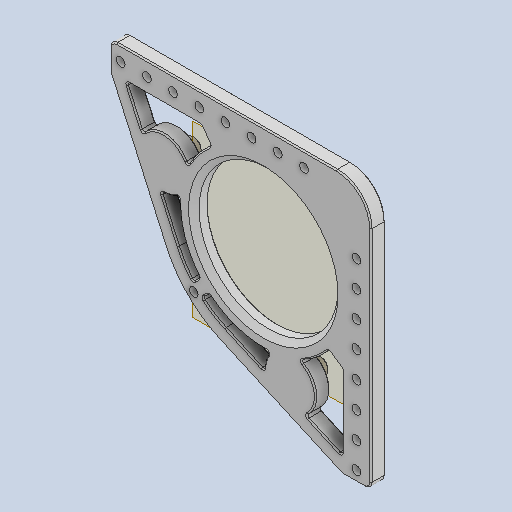
# Autodesk Inventor part: lower_plate
Saved by Autodesk Inventor 2022 (Build 260153000, 153)
## iProperties
Created: 2022-03-16
Part Number: lower_plate
Material: Generic
Document SubType Name: Modeling
Designer: zac-h
Density: 1 g/cm^3
Appearance: Default
Author: zac-h
## iProperties of the stored document lower_plate_3DPrint.ipt
Created: 2022-03-17
Part Number: lower_plate_3DPrint
Material: Generic
Document SubType Name: Modeling
Designer: zac-h
Density: 1 g/cm^3
Appearance: Default
Author: zac-h
Autodesk Inventor part; units mm, degrees
ref_plane "YZ Plane" through (0, 0, 0) normal (1, 0, 0) x (0, 1, 0)
ref_plane "XZ Plane" through (0, 0, 0) normal (0, 1, 0) x (-1, 0, 0)
ref_plane "XY Plane" through (0, 0, 0) normal (0, 0, 1) x (1, 0, 0)
ref_plane "Work Plane1" through (0, 0, 3) normal (0, 0, 1) x (1, 0, 0)
sketch "Sketch1" plane through (0, 0, 3) normal (0, 0, 1) x (1, 0, 0)
  circle A0 centre (-0.1388, 10.4389) radius 38.025 construction
  circle A1 centre (-0.1388, 10.4389) radius 33.675
  line L0 (41.1362, 10.4389) -> (-0.1388, 10.4389) construction
  circle A2 centre (-0.1388, 10.4389) radius 52.145
  line L1 (-0.1388, 62.5839) -> (-74.3588, 62.5839)
  line L2 (-74.3588, 62.5839) -> (-74.3588, 48.6139)
  line L3 (-74.3588, 48.6139) -> (-35.6602, 48.6139)
  line L4 (-74.3588, 55.5989) -> (45.0212, 55.5989) construction
  line L5 (45.0212, 55.5989) -> (-0.1388, 10.4389) construction
  circle A3 centre (-31.1788, 55.5989) radius 2.132
  circle A4 centre (-43.8788, 55.5989) radius 2.132
  circle A5 centre (-56.5788, 55.5989) radius 2.132
  circle A6 centre (-69.2788, 55.5989) radius 2.132
  line L6 (52.0062, 10.4389) -> (52.0062, -63.7811)
  line L7 (52.0062, -63.7811) -> (38.0362, -63.7811)
  line L8 (38.0362, -63.7811) -> (38.0362, -25.0825)
  circle A7 centre (45.0212, -20.6011) radius 2.132
  circle A8 centre (45.0212, -33.3011) radius 2.132
  circle A9 centre (45.0212, -46.0011) radius 2.132
  circle A10 centre (45.0212, -58.7011) radius 2.132
  line L9 (-47.7328, -10.8663) -> (-74.3588, 48.6139)
  line L10 (-21.444, -37.1551) -> (38.0362, -63.7811)
  circle A11 centre (-0.1388, 10.4389) radius 38.175 construction
  circle A12 centre (35.3403, 45.9179) radius 12 construction
  circle A13 centre (35.3403, 45.9179) radius 15
  line L11 (35.3403, 62.5839) -> (-0.1388, 62.5839)
  circle A14 centre (35.3403, 45.9179) radius 3.95
  circle A15 centre (-18.4788, 55.5989) radius 2.132
  circle A16 centre (-5.7788, 55.5989) radius 2.132
  circle A17 centre (6.9212, 55.5989) radius 2.132
  circle A18 centre (19.6212, 55.5989) radius 2.132
  circle A19 centre (45.0212, -7.9011) radius 2.132
  circle A20 centre (45.0212, 4.7989) radius 2.132
  circle A21 centre (45.0212, 17.4989) radius 2.132
  circle A22 centre (45.0212, 30.1989) radius 2.132
  circle A23 centre (35.3403, 45.9179) radius 16.6659
  line L12 (-35.6602, 48.6139) -> (12.0833, 48.6139) construction
  line L13 (52.0062, 45.9179) -> (52.0062, 10.4389)
  circle A24 centre (-33.8359, -23.2582) radius 2.132
  line L14 (-33.8359, -23.2582) -> (-37.0109, -26.4332) construction
  point P0 (0, 0)
  point P1 (24.5699, 56.3582)
  point P2 (45.7805, 35.1475)
  dimension "d0" = 4.35
  dimension "d11" = 13.97
  dimension "d12" = 45
  dimension "d13" = 4.264
  dimension "d14" = 76.2
  dimension "d17" = 12.7
  dimension "d23" = 119.38
  dimension "d47" = 0.15
  dimension "d48" = 24
  dimension "d49" = 30
  dimension "d50" = 7.9
  dimension "d91" = 12.7
  dimension "d96" = 4.264
  dimension "d99" = 3.175
  constraints: 30 end point, 24 centre point, 12 symmetric about line, 8 point on circle, 7 horizontal, 7 tangent, 5 coincident, 3 point on line, 2 perpendicular, 1 collinear, 1 midpoint, 22 other
  measures "d0" radial gap between concentric circles of A0 A1
  measures "d11" distance of L1.end L2.end
  measures "d12" angle of L0 L5
  measures "d13" diameter of A3
  measures "d14" distance of A3.centre L4.end
  measures "d17" distance of A3.centre A4.centre
  measures "d23" distance of L4.start L4.end
  measures "d47" radial gap between concentric circles of A0 A11
  measures "d48" diameter of A12
  measures "d49" diameter of A13
  measures "d50" diameter of A14
  measures "d91" distance of A3.centre A15.centre
  measures "d96" diameter of A24
  measures "d99" horizontal distance of L14.start L14.end
extrude "Extrusion1" add sketch "Sketch1" along normal blind 7 contours A1 A23 A22 A2 A18 | A1 A23 A18 A2 A13 A22 | A23 L13 A2 | A2 A13 A23 | A2 L11 A23 | L6 L7 L8 A2 | A13 A2 A14 | A2 A14 A13 | A2 L3 L2 L1 | L8 L10 A2 | A14 A2 | A2 A14 | A2 L9 L3
fillet "Fillet1" radius 3.175 4 edges at (38.0362, -63.7811, 6.5) (-74.3588, 48.6139, 6.5) (52.0062, -63.7811, 6.5) (-74.3588, 62.5839, 6.5)
chamfer "Chamfer1" distance 2.54 angle 45 1 edges at (-33.8138, 10.4389, 10)
chamfer "Chamfer2" distance 0.6 angle 45 1 edges at (-33.8138, 10.4389, 3)
chamfer "Chamfer3" distance 0.6 angle 45 22 edges at (7.9866, -50.3296, 3) (38.0512, -63.7111, 3) (51.0763, -62.8512, 3) (43.7728, -63.7811, 3) (52.0062, -7.3441, 3) (-37.0109, -26.4332, 3) (-17.9217, 62.5839, 3) (-73.4288, 61.6539, 3) (-74.3588, 54.3505, 3) (-74.2887, 48.6288, 3) (-60.9072, 18.5642, 3) (7.9866, -50.3296, 10) (38.0512, -63.7111, 10) (51.0763, -62.8512, 10) (43.7728, -63.7811, 10) (52.0062, -7.3441, 10) (-37.0109, -26.4332, 10) (-17.9217, 62.5839, 10) (-73.4288, 61.6539, 10) (-74.3588, 54.3505, 10) (-74.2887, 48.6288, 10) (-60.9072, 18.5642, 10)
sketch "Sketch4" plane through (0, 0, 3) normal (0, 0, -1) x (-1, 0, 0)
  circle A0 centre (-35.3403, 45.9179) radius 3.95 projected
  point P0 (0, 0)
extrude "Extrusion4" add sketch "Sketch4" along normal blind 8
sketch "Sketch5" plane through (0, 0, 3) normal (0, 0, -1) x (-1, 0, 0)
  circle A0 centre (-35.3403, 45.9179) radius 3.95 projected
  circle A1 centre (-35.3403, 45.9179) radius 6.05
  point P0 (0, 0)
  dimension "d53" = 12.1
  constraints: 1 centre point, 1 coincident
  measures "d53" diameter of A1
extrude "Extrusion5" add sketch "Sketch5" along normal blind 3
chamfer "Chamfer5" distance 0.6 angle 45 1 edges at (39.2903, 45.9179, -5)
pattern_circular "Circular Pattern1" count 3 over 360 about axis through (-0.1388, 10.4389, 3) along (0, 0, 1) of "Extrusion5", "Extrusion4", "Chamfer5"
sketch "Sketch6" plane through (0, 0, 3) normal (0, 0, -1) x (-1, 0, 0)
  circle A0 centre (-12.8475, -38.0265) radius 6.05 projected
  circle A1 centre (48.6041, 23.4251) radius 6.05 projected
  circle A2 centre (-35.3403, 45.9179) radius 6.05 projected
  circle A3 centre (0.1388, 10.4389) radius 34.275 projected
  circle A4 centre (31.1788, 55.5989) radius 2.132 projected
  circle A5 centre (43.8788, 55.5989) radius 2.132 projected
  circle A6 centre (56.5788, 55.5989) radius 2.132 projected
  circle A7 centre (69.2788, 55.5989) radius 2.132 projected
  circle A8 centre (-45.0212, -33.3011) radius 2.132 projected
  circle A9 centre (-45.0212, -46.0011) radius 2.132 projected
  circle A10 centre (-45.0212, -58.7011) radius 2.132 projected
  circle A11 centre (-45.0212, -20.6011) radius 2.132 projected
  line L0 (21.1988, -36.6075) -> (-37.6624, -62.9564) projected
  arc A12 (21.1988, -36.6075) -> (47.1851, -10.6212) centre (0.1388, 10.4389) ccw projected
  line L1 (73.534, 48.24) -> (47.1851, -10.6212) projected
  arc A13 (73.534, 48.24) -> (73.7588, 49.2921) centre (71.1838, 49.2921) ccw projected
  line L2 (73.7588, 59.4089) -> (73.7588, 49.2921) projected
  arc A14 (73.7588, 59.4089) -> (71.1838, 61.9839) centre (71.1838, 59.4089) ccw projected
  arc A15 (-51.4062, -60.6061) -> (-48.8312, -63.1811) centre (-48.8312, -60.6061) ccw projected
  line L3 (-38.7144, -63.1811) -> (-48.8312, -63.1811) projected
  arc A16 (-38.7144, -63.1811) -> (-37.6624, -62.9564) centre (-38.7144, -60.6061) ccw projected
  arc A17 (18.6044, -30.8117) -> (41.3893, -8.0267) centre (0.1388, 10.4389) ccw
  line L4 (18.6044, -30.8117) -> (-39.5208, -56.8311)
  line L5 (-39.5208, -56.8311) -> (-45.0562, -56.8311)
  line L6 (-45.0562, -56.8311) -> (-45.0562, 49.6033)
  arc A18 (35.2643, 55.6339) -> (-45.0562, 49.6033) centre (-4.896, 52.6186) ccw
  line L7 (35.2643, 55.6339) -> (67.4088, 55.6339)
  line L8 (67.4088, 55.6339) -> (67.4088, 50.0984)
  line L9 (67.4088, 50.0984) -> (41.3893, -8.0267)
  circle A19 centre (48.6041, 23.4251) radius 12.4
  circle A20 centre (-12.8475, -38.0265) radius 12.4
  circle A21 centre (-35.3403, 45.9179) radius 12.4
  circle A22 centre (0.1388, 10.4389) radius 40.625
  circle A23 centre (69.2788, 55.5989) radius 2.132 projected
  circle A24 centre (31.1788, 55.5989) radius 2.132 projected
  line L10 (69.2788, 55.5989) -> (31.1788, 55.5989) construction
  line L11 (69.2788, 62.5839) -> (31.1788, 62.5839)
  line L12 (31.1788, 48.6139) -> (69.2788, 48.6139)
  arc A25 (69.2788, 48.6139) -> (69.2788, 62.5839) centre (69.2788, 55.5989) ccw
  arc A26 (31.1788, 62.5839) -> (31.1788, 48.6139) centre (31.1788, 55.5989) ccw
  circle A27 centre (-45.0212, -58.7011) radius 2.132 projected
  circle A28 centre (-45.0212, -20.6011) radius 2.132 projected
  line L13 (-45.0212, -58.7011) -> (-45.0212, -20.6011) construction
  line L14 (-38.0362, -58.7011) -> (-38.0362, -20.6011)
  line L15 (-52.0062, -20.6011) -> (-52.0062, -58.7011)
  arc A29 (-52.0062, -58.7011) -> (-38.0362, -58.7011) centre (-45.0212, -58.7011) ccw
  arc A30 (-38.0362, -20.6011) -> (-52.0062, -20.6011) centre (-45.0212, -20.6011) ccw
  line L16 (0.1388, 10.4389) -> (-45.0212, -20.6011) construction
  line L17 (-1.6597, 13.0554) -> (-46.8197, -17.9846)
  line L18 (-43.2228, -23.2177) -> (1.9372, 7.8223)
  arc A31 (1.9372, 7.8223) -> (-1.6597, 13.0554) centre (0.1388, 10.4389) ccw
  arc A32 (-46.8197, -17.9846) -> (-43.2228, -23.2177) centre (-45.0212, -20.6011) ccw
  line L19 (31.1788, 55.5989) -> (0.1388, 10.4389) construction
  line L20 (28.5622, 57.3973) -> (-2.4778, 12.2373)
  line L21 (2.7553, 8.6404) -> (33.7953, 53.8004)
  arc A33 (33.7953, 53.8004) -> (28.5622, 57.3973) centre (31.1788, 55.5989) ccw
  arc A34 (-2.4778, 12.2373) -> (2.7553, 8.6404) centre (0.1388, 10.4389) ccw
  line L22 (0.1388, 10.4389) -> (37.0109, -26.4332) construction
  arc A35 (21.444, -37.1551) -> (47.7328, -10.8663) centre (0.1388, 10.4389) ccw projected
  line L23 (-2.1063, 8.1938) -> (34.7658, -28.6783)
  line L24 (39.2559, -24.1882) -> (2.3838, 12.6839)
  arc A36 (2.3838, 12.6839) -> (-2.1063, 8.1938) centre (0.1388, 10.4389) ccw
  arc A37 (34.7658, -28.6783) -> (39.2559, -24.1882) centre (37.0109, -26.4332) ccw
  line L25 (0.1388, 10.4389) -> (52.2838, 10.4389) construction
  line L26 (-35.3403, 61.9839) -> (71.1838, 61.9839) projected
  arc A38 (-35.3403, 61.9839) -> (-51.4062, 45.9179) centre (-35.3403, 45.9179) ccw projected
  line L27 (-51.4062, -60.6061) -> (-51.4062, 45.9179) projected
  point P0 (0, 0)
  point P1 (50.2288, 55.5989)
  point P2 (-45.0212, -39.6511)
  point P3 (-22.4412, -5.0811)
  point P4 (15.6588, 33.0189)
  point P5 (18.5748, -7.9972)
  point P6 (31.0222, -15.9544)
  point P7 (34.2626, -19.1948)
  point P8 (49.9506, 11.0984)
  point P9 (40.6123, 13.944)
  point P10 (29.7724, -23.6849)
  point P11 (26.5321, -20.4446)
  point P12 (-3.3664, -30.0346)
  point P13 (-0.5208, -39.373)
  point P14 (-41.6923, -14.4604)
  point P15 (-35.0366, -9.8857)
  point P16 (-33.1597, 33.7112)
  point P17 (-45.0562, 38.2133)
  point P18 (-45.0562, -13.6162)
  point P19 (-31.4397, -15.1188)
  point P20 (-38.0955, -19.6935)
  point P21 (-38.0362, -56.1666)
  point P22 (-20.0544, -48.1171)
  point P23 (-17.0624, -26.3648)
  point P24 (30.2711, 48.6731)
  point P25 (25.6964, 42.0173)
  point P26 (36.9424, 27.64)
  point P27 (58.6947, 30.632)
  point P28 (66.7442, 48.6139)
  point P29 (20.4633, 45.6142)
  point P30 (25.038, 52.27)
  point P31 (24.1939, 55.6339)
  point P32 (-25.555, 53.6144)
  point P33 (-23.1335, 43.7374)
  dimension "d62" = 6.35
  dimension "d63" = 6.35
  dimension "d64" = 6.35
  dimension "d65" = 13.97
  dimension "d66" = 13.97
  dimension "d67" = 6.35
  dimension "d68" = 6.35
  dimension "d69" = 45
  dimension "d70" = 6.35
  constraints: 54 end point, 25 point on circle, 20 tangent, 16 centre point, 5 midpoint, 5 parallel, 3 equal radius, 2 horizontal, 1 equal length, 1 perpendicular, 3 other
  measures "d62" distance between parallel lines of L1 L9
  measures "d63" radial gap between concentric circles of A1 A19
  measures "d64" radial gap between concentric circles of A3 A22
  measures "d65" diameter of A26
  measures "d66" diameter of A30
  measures "d67" diameter of A32
  measures "d68" diameter of A34
  measures "d69" angle of L22 L25
  measures "d70" diameter of A37
extrude "Extrusion6" cut sketch "Sketch6" against normal through all contours L21 A26 L12 L9 A19 A22 | A22 A19 L9 A17 L24 | L23 A17 L4 A20 A22 | A22 A20 L4 L14 A30 L18
fillet "Fillet3" radius 1 18 edges at (17.0624, -26.3648, 6.5) (31.4397, -15.1188, 6.5) (38.0955, -19.6935, 6.5) (38.0362, -56.1666, 6.5) (20.0544, -48.1171, 6.5) (-31.0222, -15.9544, 6.5) (-34.2626, -19.1948, 6.5) (-49.9506, 11.0984, 6.5) (-40.6123, 13.944, 6.5) (-30.2711, 48.6731, 6.5) (-25.6964, 42.0173, 6.5) (-36.9424, 27.64, 6.5) (-58.6947, 30.632, 6.5) (-66.7442, 48.6139, 6.5) (-29.7724, -23.6849, 6.5) (-26.5321, -20.4446, 6.5) (3.3664, -30.0346, 6.5) (0.5208, -39.373, 6.5)
chamfer "Chamfer6" distance 0.6 angle 45 80 edges at (-47.1388, 35.7382, 3) (-36.8934, 28.9571, 3) (-31.7761, 35.9236, 3) (-26.0472, 42.0718, 3) (-28.0771, 45.481, 3) (-30.3215, 48.5214, 3) (-30.9973, 48.6162, 3) (-48.1899, 48.6139, 3) (-66.0402, 48.1577, 3) (-62.7354, 39.6586, 3) (-58.6064, 31.5337, 3) (-47.1388, 35.7382, 10) (-58.6064, 31.5337, 10) (-62.7354, 39.6586, 10) (-66.0402, 48.1577, 10) (-48.1899, 48.6139, 10) (-30.9973, 48.6162, 10) (-30.3215, 48.5214, 10) (-28.0771, 45.481, 10) (-26.0472, 42.0718, 10) (-31.7761, 35.9236, 10) (-36.8934, 28.9571, 10) (-26.5217, -20.7995, 10) (2.2012, -30.6507, 10) (-41.2284, 12.7789, 10) (-31.3771, -15.9441, 10) (18.3795, -26.3158, 10) (31.4942, -15.4696, 10) (-13.0988, -28.0635, 10) (-38.6411, -2.5212, 10) (25.346, -21.1985, 10) (-29.2963, -23.6714, 10) (-0.014, -38.6416, 10) (-49.2192, 10.5637, 10) (-34.2491, -18.7187, 10) (20.9561, -48.0287, 10) (37.9438, -19.7438, 10) (37.58, -55.4625, 10) (-13.0988, -28.0635, 3) (-38.6411, -2.5212, 3) (25.346, -21.1985, 3) (-26.5217, -20.7995, 3) (2.2012, -30.6507, 3) (-41.2284, 12.7789, 3) (-31.3771, -15.9441, 3) (18.3795, -26.3158, 3) (31.4942, -15.4696, 3) (-29.2963, -23.6714, 3) (-0.014, -38.6416, 3) (-49.2192, 10.5637, 3) (-34.2491, -18.7187, 3) (20.9561, -48.0287, 3) (37.9438, -19.7438, 3) (37.58, -55.4625, 3) (38.0386, -20.4196, 10) (38.0386, -20.4196, 3) (-32.5817, -17.5139, 10) (-45.2066, 11.4996, 10) (-45.3387, 0.7959, 10) (-38.53, -13.4087, 10) (-38.53, -13.4087, 3) (-45.3387, 0.7959, 3) (-45.2066, 11.4996, 3) (-32.5817, -17.5139, 3) (0.922, -34.629, 10) (-28.0916, -22.0041, 10) (-23.9863, -27.9523, 10) (-9.7818, -34.7611, 10) (-9.7818, -34.7611, 3) (-23.9863, -27.9523, 3) (-28.0916, -22.0041, 3) (0.922, -34.629, 3) (38.0362, -37.6122, 10) (29.081, -52.1578, 10) (25.1606, -36.5611, 10) (34.9033, -17.4994, 10) (38.0362, -37.6122, 3) (34.9033, -17.4994, 3) (25.1606, -36.5611, 3) (29.081, -52.1578, 3)
body "Solid1"
